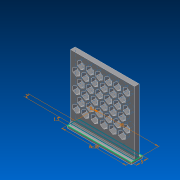
# Autodesk Inventor part: vent test hex
Saved by Autodesk Inventor 2015 (Build 190159000, 159)
## iProperties
Created: 2017-03-16
Part Number: vent test hex
Material: Generic
Document SubType Name: Modeling
Designer: ZigZagJoe
Density: 1 g/cm^3
Appearance: Default
Author: ZigZagJoe
Autodesk Inventor part; units mm, degrees
ref_plane "YZ Plane" through (0, 0, 0) normal (1, 0, 0) x (0, 1, 0)
ref_plane "XZ Plane" through (0, 0, 0) normal (0, 1, 0) x (-1, 0, 0)
ref_plane "XY Plane" through (0, 0, 0) normal (0, 0, 1) x (1, 0, 0)
sketch "Sketch1" plane through (0, 0, 0) normal (0, 0, 1) x (1, 0, 0)
  line L0 (-19.4684, -0.3877) -> (8.5316, -0.3877)
  line L1 (8.5316, -0.3877) -> (8.5316, -5.3877)
  line L2 (8.5316, -5.3877) -> (-19.4684, -5.3877)
  line L3 (-19.4684, -5.3877) -> (-19.4684, -0.3877)
  line L4 (-19.4684, -1.8877) -> (8.5316, -1.8877)
  line L5 (8.5316, -1.8877) -> (8.5316, -3.8877)
  line L6 (8.5316, -3.8877) -> (-19.4684, -3.8877)
  line L7 (-19.4684, -3.8877) -> (-19.4684, -1.8877)
  point P0 (0, 0)
  dimension "d0" = 28
  dimension "d1" = 5
  dimension "d4" = 2
  dimension "d5" = 28
  dimension "d7" = 1.5
  dimension "d56" = 0
  constraints: 16 end point, 4 parallel, 2 horizontal, 2 perpendicular
  measures "d0" distance of L1.end L2.end
  measures "d1" distance of L0.end L1.end
  measures "d4" distance of L6.end L4.start
  measures "d5" distance of L4.start L4.end
  measures "d7" distance between parallel lines of L2 L6
  measures "d56" distance between parallel lines of L3 L7
extrude "Extrusion1" add sketch "Sketch1" along normal blind 28 contours L4 L1 L6 L3
extrude "Extrusion2" add sketch "Sketch1" against normal blind 1
fillet "Fillet1" radius 1 2 edges at (-5.4684, -3.8877, 0) (-5.4684, -1.8877, 0)
sketch "Sketch2" plane through (-19.4684, -3.8877, 28) normal (0, -1, 0) x (1, 0, 0)
  line L0 (27, -1) -> (1, -1)
  line L1 (1, -1) -> (1, -17)
  line L2 (1, -17) -> (27, -17)
  line L3 (27, -17) -> (27, -1)
  line L4 (0, 0) -> (28, 0) projected
  line L5 (2.3536, -1) -> (7.3536, -1) construction
  line L6 (8.0711, -1) -> (5.2426, -3.8284)
  line L7 (5.2426, -3.8284) -> (2.4142, -1)
  line L8 (1, -2.4142) -> (3.8284, -5.2426)
  line L9 (3.8284, -5.2426) -> (1, -8.0711)
  line L10 (1, -8.0711) -> (2.4142, -9.4853)
  line L11 (2.4142, -9.4853) -> (5.2426, -6.6569)
  line L12 (5.2426, -6.6569) -> (8.0711, -9.4853)
  line L13 (8.0711, -9.4853) -> (9.4853, -8.0711)
  line L14 (9.4853, -8.0711) -> (6.6569, -5.2426)
  line L15 (6.6569, -5.2426) -> (9.4853, -2.4142)
  line L16 (9.4853, -2.4142) -> (8.0711, -1)
  line L17 (2.4142, -1) -> (1, -2.4142)
  line L18 (9.4853, -2.4142) -> (9.4853, -8.0711)
  line L19 (8.0711, -9.4853) -> (2.4142, -9.4853)
  line L20 (1, -8.0711) -> (1, -2.4142)
  line L21 (2.4142, -1) -> (8.0711, -1)
  line L22 (28, -27) -> (28, 0) projected
  line L23 (0, -27) -> (0, 0) projected
  point P0 (19.4684, -28)
  dimension "d28" = 4
  dimension "d29" = 2
  dimension "d30" = 4
  dimension "d31" = 2
  dimension "d32" = 4
  dimension "d39" = 8.4853
  dimension "d40" = 1
  dimension "d41" = 1
  dimension "d42" = 1
  constraints: 42 end point, 12 point on line, 7 perpendicular, 4 parallel, 2 horizontal, 1 collinear
  measures "d28" distance of L11.end L12.end
  measures "d29" distance of L12.end L13.end
  measures "d30" distance of L14.end L15.end
  measures "d31" distance between parallel lines of L11 L9
  measures "d32" distance of L8.start L8.end
  measures "d39" horizontal distance of L13.end L8.start
  measures "d40" distance between parallel lines of L22 L3
  measures "d41" distance between parallel lines of L23 L20
  measures "d42" distance between parallel lines of L4 L0
extrude "Extrusion3" [suppressed]
pattern_linear "Rectangular Pattern1" [suppressed]
sketch "Sketch3" plane through (-19.4684, -3.8877, 28) normal (0, -1, 0) x (1, 0, 0)
  line L0 (3, -3) -> (3, -21) construction
  line L1 (2, -3) -> (2, -21)
  line L2 (4, -21) -> (4, -3)
  arc A0 (4, -3) -> (2, -3) centre (3, -3) ccw
  arc A1 (2, -21) -> (4, -21) centre (3, -21) ccw
  line L3 (0, 0) -> (28, 0) projected
  line L4 (0, -27) -> (0, 0) projected
  point P0 (19.4684, -28)
  point P1 (3, -12)
  dimension "d43" = 2
  dimension "d44" = 3
  dimension "d45" = 18
  dimension "d48" = 3
  constraints: 8 end point, 4 point on circle, 4 tangent, 2 centre point, 1 midpoint, 1 parallel, 1 vertical
  measures "d43" diameter of A1
  measures "d44" distance from line of L0.start L3
  measures "d45" distance of L0.start L0.end
  measures "d48" distance from line of L4 L0.start
extrude "Extrusion4" [suppressed]
pattern_linear "Rectangular Pattern2" [suppressed]
fillet "Fillet2" [suppressed]
sketch "Sketch4" plane through (-19.4684, -3.8877, 28) normal (0, -1, 0) x (1, 0, 0)
  line L0 (4.5, -2) -> (6, -2.866)
  line L1 (6, -2.866) -> (6, -4.5981)
  line L2 (6, -4.5981) -> (4.5, -5.4641)
  line L3 (4.5, -5.4641) -> (3, -4.5981)
  line L4 (3, -4.5981) -> (3, -2.866)
  line L5 (3, -2.866) -> (4.5, -2)
  line L6 (0, -27) -> (0, 0) projected
  line L7 (4, -8.0622) -> (2.5, -8.9282)
  line L8 (2.5, -8.9282) -> (1, -8.0622)
  line L9 (1, -8.0622) -> (1, -6.3301)
  line L10 (1, -6.3301) -> (2.5, -5.4641)
  line L11 (2.5, -5.4641) -> (4, -6.3301)
  line L12 (4, -6.3301) -> (4, -8.0622)
  line L13 (8, -8.0622) -> (6.5, -8.9282)
  line L14 (6.5, -8.9282) -> (5, -8.0622)
  line L15 (5, -8.0622) -> (5, -6.3301)
  line L16 (5, -6.3301) -> (6.5, -5.4641)
  line L17 (6.5, -5.4641) -> (8, -6.3301)
  line L18 (8, -6.3301) -> (8, -8.0622)
  line L19 (10, -2.866) -> (10, -4.5981)
  line L20 (10, -4.5981) -> (8.5, -5.4641)
  line L21 (8.5, -5.4641) -> (7, -4.5981)
  line L22 (7, -4.5981) -> (7, -2.866)
  line L23 (7, -2.866) -> (8.5, -2)
  line L24 (8.5, -2) -> (10, -2.866)
  point P0 (19.4684, -28)
  point P1 (4.5, -3.7321)
  point P2 (2.5, -7.1962)
  point P3 (6.5, -7.1962)
  point P4 (8.5, -3.7321)
  dimension "d57" = 3
  dimension "d58" = 2
  dimension "d59" = 3
  dimension "d62" = 0
  dimension "d63" = 3
  dimension "d64" = 1
  dimension "d65" = 0.5
  dimension "d67" = 1
  dimension "d68" = 1
  dimension "d69" = 3
  dimension "d71" = 3
  dimension "d72" = 1
  dimension "d73" = 1
  constraints: 48 end point, 52 other
  measures "d57" distance between parallel lines of L6 L4
  measures "d58" vertical distance of L6.end L0.start
  measures "d59" distance between parallel lines of L5 L2
  measures "d62" angle of L6 L9
  measures "d63" distance between parallel lines of L7 L10
  measures "d64" distance of L3.end L10.end
  measures "d65" horizontal distance of L11.end L2.end
  measures "d67" distance between parallel lines of L15 L12
  measures "d68" distance of L1.end L16.end
  measures "d69" distance between parallel lines of L13 L16
  measures "d71" distance between parallel lines of L20 L23
  measures "d72" distance between parallel lines of L21 L17
  measures "d73" distance of L22.end L0.end
extrude "Extrusion5" cut sketch "Sketch4" against normal blind 10
pattern_linear "Rectangular Pattern3" count 3 spacing 8 along (1, 0, 0) count 3 spacing 7 along (0, 0, -1) of "Extrusion5"
equation "\"d0\" = d5"
equation "\"d28\" = d32"
equation "\"d29\" = d31"
equation "\"d30\" = d32"
body "Solid1"
